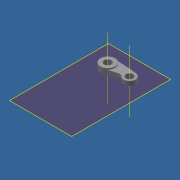
# Autodesk Inventor part: Hebel_Basis 2
Saved by Autodesk Inventor 2016 (Build 200138000, 138)
## iProperties
Created: 2014-12-22
Part Number: Hebel_Basis 2
Material: Generisch
Document SubType Name: Modeling
Designer: 4ndreas
Density: 1 g/cm^3
Appearance: Vorgabe
Mass: 0.565836 g
Surface Area: 6.0669 cm^2
Volume: 0.565836 cm^3
Author: 4ndreas
Autodesk Inventor part; units mm, degrees
ref_plane "YZ Plane" through (0, 0, 0) normal (1, 0, 0) x (0, 1, 0)
ref_plane "XZ Plane" through (0, 0, 0) normal (0, 1, 0) x (-1, 0, 0)
ref_plane "XY Plane" through (0, 0, 0) normal (0, 0, 1) x (1, 0, 0)
sketch "Skizze1" plane through (0, 0, 0) normal (0, 0, 1) x (1, 0, 0)
  line L0 (0, 0) -> (15, 0) construction
  arc A0 (0, 5) -> (3.0095, -3.9929) centre (0, 0) ccw
  arc A1 (11.376, -1.693) -> (15.531, 3.9646) centre (15, 0) ccw
  arc A2 (15.531, 3.9646) -> (0, 5) centre (0, -112) ccw
  arc A3 (11.376, -1.693) -> (3.0095, -3.9929) centre (19.3309, -47.0001) ccw
  line L1 (0, -0.0371) -> (0, 5) construction
  dimension "d0" = 15
  dimension "d1" = 5
  dimension "d2" = 1
  dimension "d3" = 4
  constraints: 8 point on circle, 4 centre point, 4 end point, 2 coincident, 2 tangent, 1 horizontal, 1 perpendicular, 1 point on line
  measures "d0" distance of L0.start L0.end
  measures "d1" radius of A0
  measures "d2" distance edge to line of A3 L0
  measures "d3" radius of A1
ref_plane "Arbeitsebene1" through (0, -0.0371, 0) normal (0, 0, -1) x (0, 1, 0)
extrude "Extrusion1" add sketch "Skizze1" along normal blind 3
sketch "Skizze2" plane through (0, 0, 3) normal (0, 0, 1) x (1, 0, 0)
  arc A0 (0, 5) -> (3.0095, -3.9929) centre (0, 0) ccw projected
  arc A1 (11.376, -1.693) -> (15.531, 3.9646) centre (15, 0) ccw projected
hole "Bohrung1" at (0, 0, 3) at (15, 0, 3) direction (0, 0, -1) diameter 3 end through all
sketch "Skizze4" plane through (0, 0, 3) normal (0, 0, 1) x (1, 0, 0)
  arc A0 (0, 5) -> (3.0095, -3.9929) centre (0, 0) ccw projected
  circle A1 centre (0, 0) radius 5
  circle A2 centre (0, 0) radius 1.5 projected
  constraints: 1 centre point, 1 coincident, 1 concentric
extrude "Extrusion2" add sketch "Skizze4" along normal blind 0.8
fillet "Rundung2" radius 2 2 edges at (3.0095, -3.9929, 1.5) (11.376, -1.693, 1.5)
sketch "Skizze3" plane through (0, 0, 0) normal (0, 0, -1) x (-1, 0, 0)
  circle A0 centre (-4.319, 1.2636) radius 1.5
  arc A1 (-3.0095, -3.9929) -> (0, 5) centre (0, 0) ccw projected
  line L0 (0, 0) -> (-4.319, 1.2636)
  circle A2 centre (0, 0) radius 4.5 construction
  dimension "d25" = 9
  constraints: 2 coincident, 2 end point, 1 centre point, 3 other
equation "\"d0\" = Hebel_basis_2"
equation "\"d3\" = bearingWall"
equation "\"d6\" = bearingHole"
equation "\"FingerLaenge_B\" = 25"
equation "\"Hebel_B\" = 25"
equation "\"FingerWall\" = 3"
equation "\"Finger_diameter\" = 8"
equation "\"Finger_width\" = 22"
equation "\"Hebel_basis_2\" = 15"
equation "\"Join_width\" = 3"
equation "\"bearingHole\" = 3"
equation "\"bearingWall\" = 4"
equation "\"support_D\" = 0.25"
